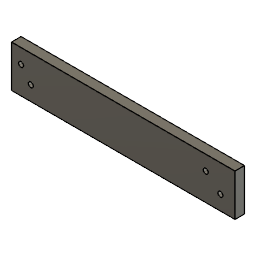
3D Printer Assembly (Autodesk Fusion 360 archive; units mm, degrees)
design "Side Panel"
Autodesk Fusion 360 part; units mm, degrees
sketch "Sketch1" plane through (0, 0, 0) normal (0, 1, 0) x (1, 0, 0)
  line L0 (0, 0) -> (-229.22, 0)
  line L1 (-229.22, 0) -> (-229.22, 10)
  line L2 (-229.22, 10) -> (0, 10)
  line L3 (0, 10) -> (0, 0)
  dimension "d1" = 10
  dimension "d2" = 229.22
  constraint coincident L0.start L3.end
  constraint horizontal L0
  constraint perpendicular L0 L1
  constraint perpendicular L1 L2
  constraint perpendicular L0 L3
  measures "d1" distance of L2.end L0.start
  measures "d2" distance of L0.start L0.end
extrude "Extrude1" add sketch "Sketch1" along normal blind 43
sketch "Sketch2" plane through (0, 0, 0) normal (0, 0, 1) x (1, 0, 0)
  line L0 (-229.22, 0) -> (0, 0)
  line L1 (0, 0) -> (0, 43)
  line L2 (0, 43) -> (-229.22, 43)
  line L3 (-229.22, 43) -> (-229.22, 0)
  point P0 (-30, 28)
  point P1 (-15, 15)
  point P2 (-219.22, 28)
  point P3 (-209.22, 15)
  dimension "d5" = 15
  dimension "d6" = 15
  dimension "d7" = 30
  dimension "d8" = 15
  dimension "d9" = 10
  dimension "d10" = 20
  dimension "d11" = 15
  dimension "d12" = 15
  measures "d5" distance of L2 P0
  measures "d6" distance of L0 P1
  measures "d7" distance of L1 P0
  measures "d8" distance of L1 P1
  measures "d9" distance of L3 P2
  measures "d10" distance of L3 P3
  measures "d11" distance of L0 P3
  measures "d12" distance of L2 P2
hole "Hole1" at (-30, 28, 0) at (-15, 15, 0) at (-219.22, 28, 0) at (-209.22, 15, 0) direction (0, 0, -1) diameter 5.105 end through all
extrude "Extrude2" cut 1 faces at (-85.2998, 17.4111, 0) along direction (0, 0, -1) blind 0.127
extrude "Extrude3" cut 1 faces at (0, 14.3333, -6.709) along direction (-1, 0, 0) blind 0.127
extrude "Extrude4" cut 1 faces at (-229.22, 14.3333, -3.418) along direction (1, 0, 0) blind 0.127

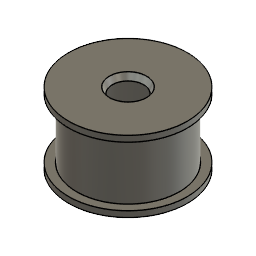
design "idler"
Autodesk Fusion 360 part; units mm, degrees
sketch "Sketch1" plane through (0, 0, 0) normal (0, 0, 1) x (1, 0, 0)
  line L0 (10, 0) -> (10, 1)
  line L1 (10, 1) -> (0, 1)
  line L2 (0, 0) -> (0, 12)
  line L3 (10, 0) -> (0, 0)
  line L4 (7.127, 0) -> (7.127, 12)
  line L5 (7.127, 12) -> (0, 12)
  line L6 (7.127, 12) -> (10, 12)
  line L7 (10, 12) -> (10, 11)
  line L8 (10, 11) -> (0, 11)
  line L9 (8.627, 11) -> (8.627, 1)
  line L10 (0, 6) -> (7.127, 6)
  line L11 (2.625, 11) -> (2.625, 1)
  line L12 (2.625, 11) -> (3.125, 12)
  line L13 (2.625, 1) -> (3.125, 0)
  dimension "d3" = 10
  dimension "d5" = 7.127
  dimension "d6" = 1.5
  dimension "d7" = 10
  dimension "d15" = 1
  dimension "d16" = 1
  dimension "d17" = 5
  dimension "d20" = 2.625
  dimension "d21" = 0.5
  dimension "d22" = 0.5
  constraint vertical L0
  constraint perpendicular L0 L1
  constraint coincident L2.start L3.end
  constraint vertical L2
  constraint perpendicular L2 L3
  constraint coincident L3 L4.start
  constraint perpendicular L3 L4
  constraint perpendicular L4 L5
  constraint perpendicular L0 L6
  constraint perpendicular L1 L7
  constraint coincident L2 L8.end
  constraint perpendicular L2 L8
  constraint coincident L8 L9.start
  constraint coincident L1 L9.end
  constraint perpendicular L1 L9
  constraint midpoint L2 L10.start
  constraint midpoint L4 L10.end
  constraint coincident L1.end L2
  constraint coincident L8 L11.start
  constraint coincident L1 L11.end
  constraint perpendicular L1 L11
  constraint coincident L5 L12.end
  constraint coincident L3 L13.end
  measures "d3" distance of L0.start L2.start
  measures "d5" distance of L2 L4
  measures "d6" distance of L4 L9
  measures "d7" distance of L2.end L6.end
  measures "d15" distance of L6.end L7.end
  measures "d16" distance of L0.start L0.end
  measures "d17" distance of L8 L10
  measures "d20" distance of L2 L11
  measures "d21" horizontal distance of L11.start L12.end
  measures "d22" horizontal distance of L11.end L13.end
revolve "Revolve2" add sketch "Sketch1" angle 360 about axis through (0, 0, 0) along (0, 1, 0) contours L0 L1 L3 L4 | L1 L3 L4 L13 | L1 L4 L8 L9 | L4 L6 L7 L8 | L4 L5 L8 L12

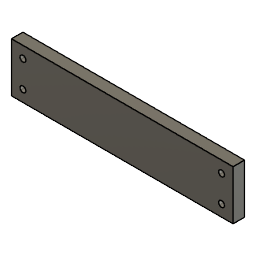
design "Back Panel"
Autodesk Fusion 360 part; units mm, degrees
sketch "Sketch1" plane through (0, 0, 0) normal (0, 1, 0) x (1, 0, 0)
  line L0 (0, 0) -> (0, 10)
  line L1 (0, 10) -> (-192.4, 10)
  line L2 (-192.4, 10) -> (-192.4, 0)
  line L3 (-192.4, 0) -> (0, 0)
  dimension "d1" = 192.4
  dimension "d2" = 10
  constraint coincident L0.start L3.end
  constraint vertical L0
  constraint perpendicular L0 L1
  constraint perpendicular L1 L2
  constraint perpendicular L0 L3
  measures "d1" distance of L2.end L0.start
  measures "d2" distance of L0.start L0.end
extrude "Extrude1" add sketch "Sketch1" along normal blind 43
sketch "Sketch2" plane through (0, 0, 0) normal (0, 0, 1) x (1, 0, 0)
  line L0 (-192.4, 0) -> (0, 0)
  line L1 (0, 0) -> (0, 43)
  line L2 (0, 43) -> (-192.4, 43)
  line L3 (-192.4, 43) -> (-192.4, 0)
  point P0 (-10, 33)
  point P1 (-10, 10)
  point P2 (-182.4, 33)
  point P3 (-182.4, 10)
  dimension "d5" = 10
  dimension "d6" = 10
  dimension "d7" = 10
  dimension "d8" = 10
  dimension "d9" = 10
  dimension "d10" = 10
  dimension "d11" = 10
  dimension "d12" = 10
  measures "d5" distance of L1 P0
  measures "d6" distance of L1 P1
  measures "d7" distance of L2 P0
  measures "d8" distance of L0 P1
  measures "d9" distance of L3 P2
  measures "d10" distance of L2 P2
  measures "d11" distance of L3 P3
  measures "d12" distance of L0 P3
hole "Hole1" at (-10, 33, 0) at (-10, 10, 0) at (-182.4, 10, 0) at (-182.4, 33, 0) direction (0, 0, -1) diameter 5.105 end through all
equation "d9 = d5"
equation "d10 = d7"
equation "d11 = d6"
equation "d12 = d8"

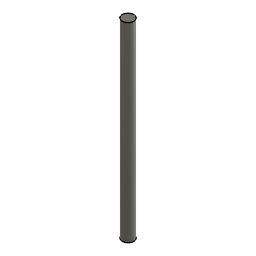
design "y-axis bars"
Autodesk Fusion 360 part; units mm, degrees
sketch "Sketch1" plane through (0, 0, 0) normal (0, 1, 0) x (1, 0, 0)
  circle A0 centre (0, 0) radius 5
  dimension "d1" = 10
  constraint coincident A0.centre origin
  measures "d1" diameter of A0
extrude "Extrude1" add sketch "Sketch1" along normal blind 162.4
